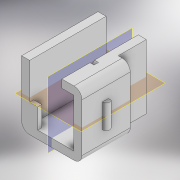
# Autodesk Inventor part: 부품1
Saved by Autodesk Inventor 2020 (Build 240168000, 168)
## iProperties
Created: 2022-04-05
Part Number: 부품1
Material: 일반
Document SubType Name: Modeling
Designer: Knowblesse
Density: 1 g/cm^3
Appearance: 기본값
Author: Knowblesse
## iProperties of the stored document _3D 인쇄.ipt
Created: 2022-04-06
Part Number: _3D 인쇄
Material: 일반
Document SubType Name: Modeling
Designer: Knowblesse
Density: 1 g/cm^3
Appearance: 기본값
Author: Knowblesse
Autodesk Inventor part; units mm, degrees
ref_plane "YZ Plane" through (0, 0, 0) normal (1, 0, 0) x (0, 1, 0)
ref_plane "XZ Plane" through (0, 0, 0) normal (0, 1, 0) x (-1, 0, 0)
ref_plane "XY Plane" through (0, 0, 0) normal (0, 0, 1) x (1, 0, 0)
sketch "스케치1" plane through (0, 0, 0) normal (0, 0, 1) x (1, 0, 0)
  line L0 (-4, -6) -> (4, -6)
  line L1 (4, -6) -> (4, 6)
  line L2 (4, 6) -> (-4, 6)
  line L3 (-4, 6) -> (-4, -6)
  line L4 (-4, -6) -> (4, 6) construction
  line L5 (4, -6) -> (-4, 6) construction
  line L6 (-6, 8) -> (-6, -8)
  line L7 (-6, -8) -> (6, -8)
  line L8 (6, -8) -> (6, 8)
  line L9 (6, 8) -> (4, 8)
  line L10 (4, 8) -> (4, 6)
  line L11 (-6, 8) -> (-4, 8)
  line L12 (-4, 8) -> (-4, 6)
  point P0 (0, 0)
  dimension "d0" = 8
  dimension "d1" = 12
  dimension "d2" = 2
  dimension "t" = 2
  dimension "d4" = 2
  dimension "d5" = 2
  constraints: 26 end point, 6 perpendicular, 2 midpoint, 2 parallel, 1 horizontal, 1 point on line, 1 vertical
  measures "d0" distance of L2.end L1.end
  measures "d1" distance of L1.end L0.end
  measures "d2" distance between parallel lines of L3 L6
  measures "t" distance between parallel lines of L8 L1
  measures "d4" distance between parallel lines of L0 L7
  measures "d5" distance between parallel lines of L11 L2
extrude "돌출1" add sketch "스케치1" along normal blind 7 contours L0 L1 L10 L9 L8 L7 L6 L11 L12 L3
sketch "스케치2" plane through (0, 0, 7) normal (0, 0, 1) x (1, 0, 0)
  line L0 (4, 8) -> (4, -6) projected
  line L1 (4, -6) -> (-4, -6) projected
  line L2 (-4, -6) -> (-4, 8) projected
  line L3 (-4, 8) -> (-6, 8) projected
  line L4 (-6, 8) -> (-6, -8) projected
  line L5 (-6, -8) -> (6, -8) projected
  line L6 (6, 8) -> (4, 8) projected
  line L7 (6, 8) -> (9, 8)
  line L8 (9, 8) -> (9, -8)
  line L9 (9, -8) -> (6, -8)
  point P0 (0, 0)
  dimension "d8" = 3
  constraints: 6 end point, 2 perpendicular, 1 horizontal
  measures "d8" distance of L8.end L5.end
extrude "돌출2" add sketch "스케치2" along normal blind 1
sketch "스케치3" plane through (0, 0, 8) normal (0, 0, 1) x (1, 0, 0)
  line L0 (-6, 8) -> (-6, -8) projected
  line L1 (-6, -8) -> (9, -8) projected
  line L2 (9, -8) -> (9, 8) projected
  line L3 (9, 8) -> (4, 8) projected
  line L4 (4, 8) -> (4, -6) projected
  line L5 (4, -6) -> (-4, -6) projected
  line L6 (-4, -6) -> (-4, 8) projected
  line L7 (-4, 8) -> (-6, 8) projected
  line L8 (4, -6) -> (-4, -6) projected
  line L9 (4, -6) -> (7, -6)
  line L10 (7, -6) -> (7, 6)
  line L11 (7, 6) -> (4, 6)
  line L12 (4, 8) -> (4, -6) projected
  point P0 (0, 0)
  point P1 (4, 6)
  dimension "d11" = 2
  dimension "d12" = 2
  constraints: 6 end point, 2 perpendicular, 1 horizontal, 1 point on line
  measures "d11" distance between parallel lines of L3 L11
  measures "d12" distance between parallel lines of L2 L10
extrude "돌출3" add sketch "스케치3" along normal blind 11 contours L7 L6 L5 L9 L10 L11 L4 L3 L2 L1 L0
sketch "스케치4" plane through (-4, -6, 0) normal (1, 0, 0) x (0, 0, -1)
  line L0 (-19, 0) -> (-19, 14) projected
  line L1 (0, 0) -> (-19, 0) projected
  line L2 (-19, 0) -> (-18, 0)
  line L3 (-18, 0) -> (-18, 5)
  line L4 (-18, 5) -> (-19, 5)
  line L5 (-19, 5) -> (-19, 0)
  point P0 (0, 6)
  dimension "d15" = 1
  dimension "d16" = 5
  constraints: 8 end point, 2 parallel, 1 horizontal, 1 perpendicular
  measures "d15" distance of L4.end L3.end
  measures "d16" distance of L3.end L2.end
extrude "돌출4" add sketch "스케치4" along normal blind 2
ref_plane "작업 평면1" through (-6, 0, 0) normal (0, 1, 0) x (1, 0, 0)
sketch "스케치5" plane through (-6, 0, 0) normal (0, 1, 0) x (1, 0, 0)
  line L0 (0, 0) -> (12, 0) projected
  line L1 (12, 0) -> (12, -7) projected
  line L2 (12, -7) -> (15, -7) projected
  line L3 (15, -7) -> (15, -19) projected
  line L4 (0, -19) -> (15, -19) projected
  line L5 (0, 0) -> (0, -19) projected
  line L6 (0, 0) -> (0, -19) projected
  circle A0 centre (0, -13) radius 0.9
  line L7 (-0.6708, -12.4) -> (0, -12.4)
  point P0 (6, 0)
  point P1 (0, -13.9)
  dimension "k" = 1.8
  dimension "d20" = 0.6
  dimension "d21" = 6
  constraints: 2 end point, 2 point on line, 1 perpendicular, 3 other
  measures "d20" distance from line of point (0, -13) L7
  measures "d21" distance from line of L4 point (0, -13)
extrude "돌출5" add sketch "스케치5" along normal mid plane 6 contours L5 A0 L7 picked at (-0.0684, -13.3921)
ref_plane "작업 평면2" through (1.5, -8, 0) normal (-1, 0, 0) x (0, 0, 1)
mirror "미러1" about plane through (1.5, -8, 0) normal (-1, 0, 0) of "돌출5"
fillet "모깎기1" radius 2 3 edges at (9, 8, 13) (-6, -8, 9.5) (9, -8, 13)
sketch "스케치6" plane through (4, 8, 0) normal (0, 1, 0) x (1, 0, 0)
  line L0 (0, 0) -> (0, -19) projected
  line L1 (0, -12) -> (1, -12)
  line L2 (1, -12) -> (1, -11.9)
  line L3 (1, -11.9) -> (0, -11.9)
  line L4 (0, -11.9) -> (0, -12)
  line L5 (3, -19) -> (0, -19) projected
  point P0 (-4, 0)
  point P1 (0, -11.9)
  dimension "d25" = 1
  dimension "d26" = 0.1
  dimension "d29" = 7
  constraints: 8 end point, 2 parallel, 1 horizontal, 1 perpendicular, 1 point on line
  measures "d25" distance of L3.end L2.end
  measures "d26" distance of L2.end L1.end
  measures "d29" distance between parallel lines of L5 L1
extrude "돌출6" cut sketch "스케치6" against normal up to surface (2 mm away)
chamfer "모따기1" distance 2 angle 45 1 edges at (4.5, 6, 12)
chamfer "모따기2" distance 1 angle 45 1 edges at (4.5, 8, 11.9)
equation "\"d2\" = t"
equation "\"d4\" = t"
equation "\"d20\" = 0.333333 * k"
